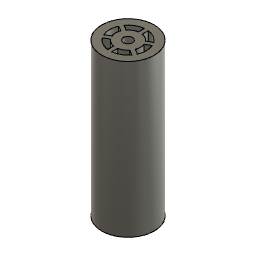
table spacer v2 (Autodesk Fusion 360 design; units mm, degrees)
Autodesk Fusion 360 part; units mm, degrees
sketch "Sketch2" plane through (0, 0, 0) normal (0, 1, 0) x (1, 0, 0)
  circle A0 centre (0, 0) radius 3.5
  circle A1 centre (0, 0) radius 9.5
  circle A2 centre (0, 0) radius 20
  circle A3 centre (0, 0) radius 14
  line L0 (0, 9.5) -> (0, 14)
  line L1 (-1.5, 13.9194) -> (-1.5, 9.3808)
  line L2 (1.5, 13.9194) -> (1.5, 9.3808)
  dimension "d5" = 7
  dimension "d6" = 6
  dimension "d7" = 40
  dimension "d8" = 6
  dimension "d11" = 1.5
  dimension "d12" = 1.5
  constraint coincident A0.centre A1.centre
  constraint concentric A0 A1
  constraint concentric A1 A2
  constraint concentric A2 A3
  constraint coincident A3 L0.end
  constraint vertical L0
  constraint coincident A3 L1.start
  constraint coincident A1 L1.end
  constraint parallel L0 L1
  constraint coincident A3 L2.start
  constraint coincident A1 L2.end
  constraint parallel L1 L2
  measures "d5" diameter of A0
  measures "d6" distance of A0 A1
  measures "d7" diameter of A2
  measures "d8" distance of A2 A3
  measures "d11" distance of L0 L2
  measures "d12" distance of L0 L1
extrude "Extrude3" add sketch "Sketch2" along normal blind 116 contours A1 A3 L0 L2 | A1 A3 L0 L1 makes body 1
extrude "Extrude2" add sketch "Sketch2" along normal blind 116 separate body contours A1 | A2 makes body 2 at (9.4528, 38.6667, 0.9459) makes body 3 at (19.9751, 77.3333, 0.9969)
pattern_circular "C-Pattern1" count 6 over 360 about axis through (0, 1.75, 0) along (0, 1, 0) of bodies 1 makes body 4 at (-9.9944, 38.6667, -7.5023) makes body 5 at (-11.4944, 38.6667, 4.9042) makes body 6 at (-1.5, 38.6667, 12.4066) makes body 7 at (9.9944, 38.6667, 7.5023) makes body 8 at (9.9944, 38.6667, -7.5023)
combine "Combine1" operation add target body 1 tool bodies 2 3 7 8 4 5 6
